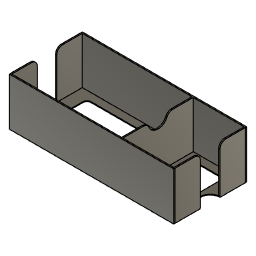
Food_Chain_Magnate_Card_Holder v1 (Autodesk Fusion 360 design; units mm, degrees)
Autodesk Fusion 360 part; units mm, degrees
sketch "Sketch1" plane through (0, 0, 0) normal (0, 0, 1) x (1, 0, 0)
  line L0 (-50, 26.6) -> (160, 26.6)
  line L1 (-50, 26.6) -> (-50, 25)
  line L2 (160, 26.6) -> (160, 25)
  line L3 (159.9999, -66.6) -> (-50, -66.6)
  line L4 (-50, -66.6) -> (-50, -65)
  line L5 (159.9999, -66.6) -> (160, -65)
  line L6 (-48.4, -64.9241) -> (-48.4, -65)
  line L7 (93.4, 25) -> (93.4, -65)
  line L8 (91.8, 25) -> (91.8, -65)
  line L9 (-48.4, 25) -> (91.8, 25)
  line L10 (93.4, 25) -> (158.4, 25)
  line L11 (158.4, -65) -> (93.4, -65)
  line L12 (91.8, -65) -> (-48.4, -65)
  line L13 (103.4, 10) -> (103.4, -50)
  line L14 (137.4, -55) -> (108.4, -55)
  line L15 (108.4, 15) -> (137.4, 15)
  line L16 (76.8, -55) -> (-27.4, -55)
  line L17 (81.8, 10) -> (81.8, -50)
  line L18 (-27.4, 15) -> (76.8, 15)
  line L19 (-32.4, 10) -> (-32.4, -50)
  line L20 (142.4, 10) -> (142.4, -50)
  arc A0 (-50, -32.5) -> (-50, -7.5) centre (-50, -20) ccw
  line L21 (-50, -65) -> (-50, -32.5)
  line L22 (-50, -7.5) -> (-50, 25)
  line L23 (-48.4, 25) -> (-48.4, -7.6028)
  line L24 (-48.4, -32.3972) -> (-48.4, -65)
  arc A1 (160, -7.5) -> (160, -32.5) centre (160, -20) ccw
  line L25 (160, 25) -> (160, -7.5)
  line L26 (160, -32.5) -> (160, -65)
  line L27 (158.4, 25) -> (158.4, -7.6028)
  line L28 (158.4, -32.3972) -> (158.4, -65)
  arc A2 (-27.4, 15) -> (-32.4, 10) centre (-27.4, 10) ccw
  arc A3 (-32.4, -50) -> (-27.4, -55) centre (-27.4, -50) ccw
  arc A4 (76.8, -55) -> (81.8, -50) centre (76.8, -50) ccw
  arc A5 (81.8, 10) -> (76.8, 15) centre (76.8, 10) ccw
  arc A6 (108.4, 15) -> (103.4, 10) centre (108.4, 10) ccw
  arc A7 (142.4, 10) -> (137.4, 15) centre (137.4, 10) ccw
  arc A8 (137.4, -55) -> (142.4, -50) centre (137.4, -50) ccw
  arc A9 (103.4, -50) -> (108.4, -55) centre (108.4, -50) ccw
  dimension "d1" = 210
  dimension "d2" = 90
  dimension "d5" = 1.6
  dimension "d6" = 1.6
  dimension "d10" = 1.6
  dimension "d11" = 1.6
  dimension "d12" = 65
  dimension "d13" = 1.6
  dimension "d16" = 16
  dimension "d17" = 16
  dimension "d18" = 25
  dimension "d19" = 25
  dimension "d24" = 5
  constraint horizontal L9
  constraint vertical L25
  constraint horizontal L11
  constraint vertical L21
  constraint perpendicular L11 L23
  constraint perpendicular L11 L27
  constraint horizontal L0
  constraint perpendicular L3 L25
  constraint coincident L6.start L23
  constraint perpendicular L6 L11
  constraint coincident L7.start L9
  constraint perpendicular L7 L11
  constraint coincident L8.end L11
  constraint perpendicular L8 L11
  constraint collinear L9 L10
  constraint collinear L11 L12
  constraint parallel L7 L13
  constraint parallel L11 L14
  constraint parallel L10 L15
  constraint parallel L12 L16
  constraint parallel L8 L17
  constraint parallel L9 L18
  constraint perpendicular L16 L19
  constraint perpendicular L14 L20
  constraint coincident A0.end L21
  constraint collinear L21 L22
  constraint coincident A0.centre L21
  constraint coincident A0 L23.end
  constraint coincident A0 L24.start
  constraint collinear L23 L24
  constraint coincident A1.end L25
  constraint collinear L25 L26
  constraint coincident A1.centre L25
  constraint coincident A1 L27.end
  constraint coincident A1 L28.start
  constraint collinear L27 L28
  constraint tangent L19 A2
  constraint tangent L18 A2
  constraint tangent L19 A3
  constraint tangent L16 A3
  constraint equal A2 A3
  constraint tangent L16 A4
  constraint tangent L17 A4
  constraint equal A2 A4
  constraint tangent L17 A5
  constraint tangent L18 A5
  constraint equal A2 A5
  constraint tangent L13 A6
  constraint tangent L15 A6
  constraint equal A2 A6
  constraint tangent L20 A7
  constraint tangent L15 A7
  constraint equal A2 A7
  constraint tangent L20 A8
  constraint tangent L14 A8
  constraint equal A2 A8
  constraint tangent L13 A9
  constraint tangent L14 A9
  constraint equal A2 A9
  measures "d1" distance of L1.end L2.end
  measures "d2" distance of L1.end L4.end
  measures "d5" distance of L21 L23
  measures "d6" distance of L25 L27
  measures "d10" distance of L0 L9
  measures "d11" distance of L3 L11
  measures "d12" distance of L7 L27
  measures "d13" distance of L7 L8
  measures "d16" distance of L19 L23
  measures "d17" distance of L20 L27
  measures "d18" diameter of A0
  measures "d19" diameter of A1
  measures "d24" radius of A2
extrude "Extrude1" add sketch "Sketch1" along normal blind 1 contours L6 L8 L9 L12 A0 L23 L24 | L7 L10 L11 A1 L27 L28 makes body 1 at (-43.0667, -49.1324, 0) makes body 2 at (153.0667, -49.1324, 0)
extrude "Extrude2" add sketch "Sketch1" along normal blind 61 contours L0 L1 L2 L3 L4 L5 L6 L7 L8 L9 L10 L11 L12 A0 L21 L22 L23 L24 A1 L25 L26 L27 L28 bodies 1 2
sketch "Sketch2" plane through (93.4, 0, 0) normal (1, 0, 0) x (0, 1, 0)
  line L0 (-65, 1) -> (25, 1)
  line L1 (25, 1) -> (25, 61)
  line L2 (25, 61) -> (-65, 61)
  line L3 (-65, 61) -> (-65, 1)
  arc A0 (-32.5, 61) -> (-7.5, 61) centre (-20, 61) ccw
  dimension "d27" = 25
  constraint midpoint L2 A0.centre
  constraint coincident L2 A0.end
  constraint coincident L2 A0.start
  measures "d27" diameter of A0
extrude "Extrude3" cut sketch "Sketch2" against normal blind 12 contours L2 A0 bodies 1
fillet "Fillet1" radius 7.5 6 edges at (-49.1983, -32.4743, 61) (-49.1983, -7.5257, 61) (159.1983, -7.5257, 61) (159.1983, -32.4743, 61) (92.6, -7.5, 61) (92.6, -32.5, 61) on bodies 1
